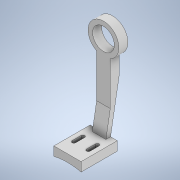
# Autodesk Inventor part: testBasePrint
Saved by Autodesk Inventor 2020.3 (Build 243373000, 373)
## iProperties
Created: 2020-06-03
Part Number: testBasePrint
Material: Generic
Document SubType Name: Modeling
Designer: robst
Density: 1 g/cm^3
Appearance: Default
Author: robst
Autodesk Inventor part; units mm, degrees
ref_plane "Work Plane3" through (19.05, 80.3219, 25.4) normal (0, 1, 0) x (-1, 0, 0)
ref_plane "Work Plane4" through (0, 228.9119, -25.0164) normal (0, 1, 0) x (-1, 0, 0)
sketch "Sketch1" plane through (0, 0, 0) normal (0, 0, 1) x (1, 0, 0)
  arc A0 (19.05, 80.3219) -> (-19.05, 80.3219) centre (0, 0) ccw
  line L0 (0, 0) -> (0, 152.4) construction
  line L1 (0, 93.0219) -> (19.05, 93.0219)
  line L2 (19.05, 93.0219) -> (19.05, 80.3219)
  line L3 (0, 93.0219) -> (-19.05, 93.0219)
  line L4 (-19.05, 93.0219) -> (-19.05, 80.3219)
  dimension "telescopeTubeDiameter" = 165.1
  dimension "d1" = 152.4
  dimension "d2" = 19.05
  dimension "d3" = 12.7
  constraints: 10 end point, 2 point on circle, 2 symmetric about line, 1 centre point, 1 coincident, 1 horizontal, 1 perpendicular, 1 point on line, 1 vertical
  measures "telescopeTubeDiameter" diameter of A0
  measures "d1" distance of L0.start L0.end
  measures "d2" distance of L1.start L1.end
  measures "d3" distance of L1.end L2.end
extrude "Extrusion1" add sketch "Sketch1" along normal mid plane 50.8
sketch "Sketch2" plane through (-19.05, 93.0219, 25.4) normal (0, 1, 0) x (1, 0, 0)
  line L0 (38.1, 0) -> (0, 0) construction
  line L1 (19.05, 0) -> (19.05, 50.8) construction
  line L2 (0, 50.8) -> (38.1, 50.8) construction
  line L3 (0, 50.8) -> (0, 0) construction
  line L4 (0, 25.4) -> (38.1, 25.4) construction
  line L5 (38.1, 50.8) -> (38.1, 0) construction
  line L6 (29.21, 19.05) -> (29.21, 31.75) construction
  line L7 (31.75, 19.05) -> (31.75, 31.75)
  line L8 (26.67, 31.75) -> (26.67, 19.05)
  arc A0 (26.67, 19.05) -> (31.75, 19.05) centre (29.21, 19.05) ccw
  arc A1 (31.75, 31.75) -> (26.67, 31.75) centre (29.21, 31.75) ccw
  point P0 (19.05, 25.4)
  point P1 (29.21, 25.4)
  dimension "d6" = 0
  dimension "d7" = 10.16
  dimension "d8" = 6.35
  dimension "d11" = 5.08
  constraints: 12 end point, 5 midpoint, 4 point on circle, 4 tangent, 2 centre point, 2 parallel
  measures "d6" distance from line of point (29.21, 25.4) L4
  measures "d7" distance between parallel lines of L6 L1
  measures "d8" distance of L6.end point (29.21, 25.4)
  measures "d11" distance between parallel lines of L7 L8
extrude "Extrusion2" cut sketch "Sketch2" against normal through all
mirror "Mirror1" about plane through (0, 0, 0) normal (1, 0, 0) of "Extrusion2"
sketch "Sketch3" plane through (0, 0, 0) normal (1, 0, 0) x (0, 1, 0)
  line L0 (93.0219, 25.4) -> (93.0219, -25.4) projected
  line L1 (80.3219, -25.4) -> (93.0219, -25.4) projected
  line L2 (162.8719, -25.4) -> (162.8719, -37.137) construction
  line L3 (93.0219, -25.4) -> (162.8719, -37.7164)
  line L4 (93.0219, -25.4) -> (162.8719, -25.4) construction
  line L5 (93.0219, -18.952) -> (162.8719, -31.2685)
  line L6 (162.8719, -31.2685) -> (162.8719, -37.7164)
  point P0 (0, 0)
  dimension "d13" = 69.85
  dimension "d14" = 10
  dimension "d15" = 6.35
  constraints: 10 end point, 2 point on line, 1 midpoint, 1 parallel, 1 perpendicular, 1 vertical
  measures "d13" distance of L0.end L2.start
  measures "d14" angle of L3 L4
  measures "d15" distance between parallel lines of L5 L3
extrude "Extrusion3" add sketch "Sketch3" along normal mid plane 19.05
ref_plane "Work Plane1" through (9.525, 162.8719, -37.7164) normal (0, 0, 1) x (1, 0, 0)
sketch "Sketch4" plane through (9.525, 162.8719, -37.7164) normal (0, 0, 1) x (1, 0, 0)
  line L0 (0, 0) -> (-19.05, 0) projected
  line L1 (-19.05, 0) -> (0, 0) construction
  line L2 (-9.525, 0) -> (-9.525, 50.8) construction
  circle A0 centre (-9.525, 44.45) radius 15.24
  arc A1 (0, 25.0747) -> (-19.05, 25.0747) centre (-9.525, 44.45) ccw
  line L3 (0, 0) -> (0, 25.0747)
  line L4 (-19.05, 0) -> (-19.05, 25.0747)
  point P0 (-9.525, -162.8719)
  dimension "d18" = 50.8
  dimension "d19" = 30.48
  dimension "d20" = 6.35
  dimension "d25" = 44.45
  constraints: 6 end point, 2 centre point, 2 point on circle, 2 vertical, 1 coincident, 1 midpoint, 1 parallel, 1 point on line
  measures "d18" distance of L2.start L2.end
  measures "d19" diameter of A0
  measures "d20" radial gap between concentric circles of A1 A0
  measures "d25" distance from line of A0.centre L0
extrude "Extrusion4" add sketch "Sketch4" along normal blind 12.7
sketch "Sketch7" plane through (0, 0, 0) normal (1, 0, 0) x (0, 1, 0)
  line L0 (93.0219, -18.952) -> (162.8719, -31.2685) projected
  line L1 (162.8719, -31.2685) -> (162.8719, -25.0164) projected
  line L2 (162.8719, -25.0164) -> (127.4148, -25.0164)
  line L3 (127.4148, -25.0164) -> (162.8719, -31.2685)
  line L4 (187.9465, -25.0164) -> (162.8719, -25.0164) projected
  line L5 (162.8719, -31.2685) -> (162.8719, -25.0164)
  point P0 (0, 0)
  constraints: 6 end point, 1 collinear, 1 horizontal, 1 point on line, 1 vertical
extrude "Extrusion5" add sketch "Sketch7" along normal mid plane 19.05
sketch "Sketch8" plane through (0, 0, 0) normal (1, 0, 0) x (0, 1, 0)
  line L0 (162.8719, 31.2685) -> (162.8719, 25.0164) projected
  line L1 (93.0219, 18.952) -> (162.8719, 31.2685) projected
  line L2 (162.8719, 25.0164) -> (127.4148, 25.0164)
  line L3 (127.4148, 25.0164) -> (162.8719, 31.2685)
  line L4 (162.8719, 31.2685) -> (162.8719, 25.0164)
  point P0 (0, 0)
  constraints: 6 end point, 1 collinear, 1 horizontal, 1 point on line
sketch "Sketch9" plane through (0, 0, 0) normal (1, 0, 0) x (0, 1, 0)
  line L0 (187.9465, 25.0164) -> (127.4148, 25.0164) projected
  line L1 (93.0219, -18.952) -> (93.0219, -25.4) projected
  line L2 (93.0219, 18.952) -> (93.0219, -18.952)
  line L3 (93.0219, -18.952) -> (127.4148, -25.0164) projected
  line L4 (93.0219, -18.952) -> (127.4148, -25.0164)
  line L5 (187.9465, -25.0164) -> (127.4148, -25.0164) projected
  line L6 (127.4148, -25.0164) -> (187.9465, -25.0164)
  line L7 (187.9465, -25.0164) -> (187.9465, 25.0164)
  line L8 (93.0219, 18.952) -> (127.4148, 25.0164) projected
  line L9 (187.9465, 25.0164) -> (127.4148, 25.0164)
  point P0 (0, 0)
  constraints: 10 end point, 2 collinear, 1 horizontal, 1 perpendicular, 1 vertical
sketch "Sketch14" plane through (0, 228.9119, -25.0164) normal (0, 1, 0) x (-1, 0, 0)
  circle A0 centre (0, -6.35) radius 2.0193
  line L0 (21.59, -12.7) -> (-21.59, -12.7) projected
  circle A1 centre (0, 56.3829) radius 2.0193
  line L1 (21.59, 62.7329) -> (-21.59, 62.7329) projected
  point P0 (0, 25.0164)
  point P1 (-9.525, -12.7)
  point P2 (9.525, -12.7)
  point P3 (-9.525, 62.7329)
  point P4 (9.525, 62.7329)
  dimension "d74" = 4.0386
  dimension "d75" = 6.35
  dimension "d76" = 6.35
  constraints: 2 centre point, 1 equal radius
  measures "d74" diameter of A0
  measures "d75" distance from line of A0.centre L0
  measures "d76" distance from line of A1.centre L1
sketch "Sketch16" plane through (0, 222.4275, -31.3664) normal (-1, 0, 0) x (0, 0, 1)
  line L0 (2.0193, 0) -> (2.0193, 6.4844)
  line L1 (2.0193, 6.4844) -> (1.4308, 6.4844)
  line L2 (1.4308, 6.4844) -> (1.4308, 0)
  line L3 (1.4308, 0) -> (2.0193, 0)
  line L4 (0, -171.8239) -> (0, 36.2042) projected
  constraints: 8 end point
sketch "Sketch15" plane through (0, 222.4275, -29.3471) normal (1, 0, 0) x (0, 1, 0)
  line L0 (-0.4631, -0.0403) -> (-0.397, -0.0403) construction
  line L1 (0.066, -0.5486) -> (-0.0001, -0.6756) construction
  line L2 (-0.7939, -0.6756) -> (-0.86, -0.5486) construction
  line L3 (-0.3308, -0.0403) -> (-0.397, 0.0868) construction
  line L4 (-0.397, 0.0868) -> (-0.4631, -0.0403) construction
  line L5 (-0.7939, -0.6756) -> (-0.7277, -0.5486) construction
  line L6 (-0.3308, -0.0403) -> (-0.0662, -0.5486)
  line L7 (-0.86, -0.5486) -> (-0.7277, -0.5486) construction
  arc A0 (-0.86, -0.5486) -> (-0.7939, -0.5887) centre (-0.7939, -0.5141) ccw construction
  line L8 (0.066, -0.5486) -> (-0.0662, -0.5486) construction
  line L9 (-0.7939, -0.6756) -> (-0.7939, -0.5486) construction
  line L10 (-0.0001, -0.6756) -> (-0.0001, -0.5486) construction
  line L11 (-0.397, 0.0868) -> (-0.397, -0.0002) construction
  line L12 (-0.7939, -0.5887) -> (-0.0001, -0.5887)
  arc A1 (-0.7939, -0.5887) -> (-0.7277, -0.5486) centre (-0.7939, -0.5141) ccw
  line L13 (-0.0662, -0.5486) -> (-0.0001, -0.6756) construction
  line L14 (-0.7277, -0.5486) -> (-0.4631, -0.0403)
  line L15 (-0.0001, -0.0002) -> (-0.0001, 0.0177)
  line L16 (-0.0001, 0.0177) -> (-0.0001, -0.0002)
  line L17 (-0.0001, -0.0002) -> (0.0334, -0.0002)
  arc A2 (-0.0662, -0.5486) -> (-0.0001, -0.5887) centre (-0.0001, -0.5141) ccw
  arc A3 (-0.0001, -0.5887) -> (0.066, -0.5486) centre (-0.0001, -0.5141) ccw construction
  arc A4 (-0.397, -0.0002) -> (-0.4631, -0.0403) centre (-0.397, -0.0747) ccw
  arc A5 (-0.3308, -0.0403) -> (-0.397, -0.0002) centre (-0.397, -0.0747) ccw
  line L18 (-0.397, -0.0002) -> (-0.397, -0.0403) construction
  line L19 (-0.397, -0.0403) -> (-0.3308, -0.0403) construction
  dimension "d94" = 55
  dimension "d95" = 0.1271
  dimension "d96" = 0.1271
  dimension "Sketch15_ThreadOffset" = 0
  dimension "Sketch15_MajorRadius" = 0.5885
  dimension "d99" = 0.7937
  dimension "Sketch15_MinorRadius" = 0
  constraints: 40 end point, 12 point on circle, 10 parallel, 8 tangent, 6 centre point, 6 collinear, 2 midpoint, 2 point on line, 1 horizontal, 1 perpendicular, 3 other
  measures "d94" angle of L6 L14
  measures "d95" distance of L3.end L0.end
  measures "d96" distance of L1.end L10.end
  measures "Sketch15_ThreadOffset" distance between parallel lines of L15 L10
  measures "Sketch15_MajorRadius" distance from line of L12 L15.start
  measures "d99" distance from line of L1.end L9
  measures "Sketch15_MinorRadius" distance edge to line of A5 L17
sketch "Sketch18" plane through (0, 222.4275, 31.3664) normal (-1, 0, 0) x (0, 0, 1)
  line L0 (2.0193, 0) -> (2.0193, 6.4844)
  line L1 (2.0193, 6.4844) -> (1.4308, 6.4844)
  line L2 (1.4308, 6.4844) -> (1.4308, 0)
  line L3 (1.4308, 0) -> (2.0193, 0)
  line L4 (0, -171.8765) -> (0, 36.5199) projected
  constraints: 8 end point
sketch "Sketch17" plane through (0, 222.4275, 33.3857) normal (1, 0, 0) x (0, 1, 0)
  line L0 (-0.4631, -0.0403) -> (-0.397, -0.0403) construction
  line L1 (0.066, -0.5486) -> (-0.0001, -0.6756) construction
  line L2 (-0.7939, -0.6756) -> (-0.86, -0.5486) construction
  line L3 (-0.3308, -0.0403) -> (-0.397, 0.0868) construction
  line L4 (-0.397, 0.0868) -> (-0.4631, -0.0403) construction
  line L5 (-0.7939, -0.6756) -> (-0.7277, -0.5486) construction
  line L6 (-0.3308, -0.0403) -> (-0.0662, -0.5486)
  line L7 (-0.86, -0.5486) -> (-0.7277, -0.5486) construction
  arc A0 (-0.86, -0.5486) -> (-0.7939, -0.5887) centre (-0.7939, -0.5141) ccw construction
  line L8 (0.066, -0.5486) -> (-0.0662, -0.5486) construction
  line L9 (-0.7939, -0.6756) -> (-0.7939, -0.5486) construction
  line L10 (-0.0001, -0.6756) -> (-0.0001, -0.5486) construction
  line L11 (-0.397, 0.0868) -> (-0.397, -0.0002) construction
  line L12 (-0.7939, -0.5887) -> (-0.0001, -0.5887)
  arc A1 (-0.7939, -0.5887) -> (-0.7277, -0.5486) centre (-0.7939, -0.5141) ccw
  line L13 (-0.0662, -0.5486) -> (-0.0001, -0.6756) construction
  line L14 (-0.7277, -0.5486) -> (-0.4631, -0.0403)
  line L15 (-0.0001, -0.0002) -> (-0.0001, 0.0177)
  line L16 (-0.0001, 0.0177) -> (-0.0001, -0.0002)
  line L17 (-0.0001, -0.0002) -> (0.0334, -0.0002)
  arc A2 (-0.0662, -0.5486) -> (-0.0001, -0.5887) centre (-0.0001, -0.5141) ccw
  arc A3 (-0.0001, -0.5887) -> (0.066, -0.5486) centre (-0.0001, -0.5141) ccw construction
  arc A4 (-0.397, -0.0002) -> (-0.4631, -0.0403) centre (-0.397, -0.0747) ccw
  arc A5 (-0.3308, -0.0403) -> (-0.397, -0.0002) centre (-0.397, -0.0747) ccw
  line L18 (-0.397, -0.0002) -> (-0.397, -0.0403) construction
  line L19 (-0.397, -0.0403) -> (-0.3308, -0.0403) construction
  dimension "d112" = 55
  dimension "d113" = 0.1271
  dimension "d114" = 0.1271
  dimension "Sketch17_ThreadOffset" = 0
  dimension "Sketch17_MajorRadius" = 0.5885
  dimension "d117" = 0.7937
  dimension "Sketch17_MinorRadius" = 0
  constraints: 40 end point, 12 point on circle, 10 parallel, 8 tangent, 6 centre point, 6 collinear, 2 midpoint, 2 point on line, 1 horizontal, 1 perpendicular, 3 other
  measures "d112" angle of L6 L14
  measures "d113" distance of L3.end L0.end
  measures "d114" distance of L1.end L10.end
  measures "Sketch17_ThreadOffset" distance between parallel lines of L15 L10
  measures "Sketch17_MajorRadius" distance from line of L12 L15.start
  measures "d117" distance from line of L1.end L9
  measures "Sketch17_MinorRadius" distance edge to line of A5 L17
sketch "Sketch20" plane through (13.0819, 199.769, -31.3664) normal (0.5, 0.866, 0) x (0, 0, 1)
  line L0 (2.0193, 0) -> (2.0193, 6.4844)
  line L1 (2.0193, 6.4844) -> (1.4308, 6.4844)
  line L2 (1.4308, 6.4844) -> (1.4308, 0)
  line L3 (1.4308, 0) -> (2.0193, 0)
  line L4 (0, -67.0949) -> (0, 89.4563) projected
  constraints: 8 end point
sketch "Sketch19" plane through (13.0819, 199.769, -29.3471) normal (-0.5, -0.866, 0) x (0.866, -0.5, 0)
  line L0 (-0.4631, -0.0403) -> (-0.397, -0.0403) construction
  line L1 (0.066, -0.5486) -> (-0.0001, -0.6756) construction
  line L2 (-0.7939, -0.6756) -> (-0.86, -0.5486) construction
  line L3 (-0.3308, -0.0403) -> (-0.397, 0.0868) construction
  line L4 (-0.397, 0.0868) -> (-0.4631, -0.0403) construction
  line L5 (-0.7939, -0.6756) -> (-0.7277, -0.5486) construction
  line L6 (-0.3308, -0.0403) -> (-0.0662, -0.5486)
  line L7 (-0.86, -0.5486) -> (-0.7277, -0.5486) construction
  arc A0 (-0.86, -0.5486) -> (-0.7939, -0.5887) centre (-0.7939, -0.5141) ccw construction
  line L8 (0.066, -0.5486) -> (-0.0662, -0.5486) construction
  line L9 (-0.7939, -0.6756) -> (-0.7939, -0.5486) construction
  line L10 (-0.0001, -0.6756) -> (-0.0001, -0.5486) construction
  line L11 (-0.397, 0.0868) -> (-0.397, -0.0002) construction
  line L12 (-0.7939, -0.5887) -> (-0.0001, -0.5887)
  arc A1 (-0.7939, -0.5887) -> (-0.7277, -0.5486) centre (-0.7939, -0.5141) ccw
  line L13 (-0.0662, -0.5486) -> (-0.0001, -0.6756) construction
  line L14 (-0.7277, -0.5486) -> (-0.4631, -0.0403)
  line L15 (-0.0001, -0.0002) -> (-0.0001, 0.0177)
  line L16 (-0.0001, 0.0177) -> (-0.0001, -0.0002)
  line L17 (-0.0001, -0.0002) -> (0.0334, -0.0002)
  arc A2 (-0.0662, -0.5486) -> (-0.0001, -0.5887) centre (-0.0001, -0.5141) ccw
  arc A3 (-0.0001, -0.5887) -> (0.066, -0.5486) centre (-0.0001, -0.5141) ccw construction
  arc A4 (-0.397, -0.0002) -> (-0.4631, -0.0403) centre (-0.397, -0.0747) ccw
  arc A5 (-0.3308, -0.0403) -> (-0.397, -0.0002) centre (-0.397, -0.0747) ccw
  line L18 (-0.397, -0.0002) -> (-0.397, -0.0403) construction
  line L19 (-0.397, -0.0403) -> (-0.3308, -0.0403) construction
  dimension "d130" = 55
  dimension "d131" = 0.1271
  dimension "d132" = 0.1271
  dimension "Sketch19_ThreadOffset" = 0
  dimension "Sketch19_MajorRadius" = 0.5885
  dimension "d135" = 0.7937
  dimension "Sketch19_MinorRadius" = 0
  constraints: 40 end point, 12 point on circle, 10 parallel, 8 tangent, 6 centre point, 6 collinear, 2 midpoint, 2 point on line, 1 horizontal, 1 perpendicular, 3 other
  measures "d130" angle of L6 L14
  measures "d131" distance of L3.end L0.end
  measures "d132" distance of L1.end L10.end
  measures "Sketch19_ThreadOffset" distance between parallel lines of L15 L10
  measures "Sketch19_MajorRadius" distance from line of L12 L15.start
  measures "d135" distance from line of L1.end L9
  measures "Sketch19_MinorRadius" distance edge to line of A5 L17
sketch "Sketch22" plane through (-13.0819, 199.769, -31.3664) normal (0.5, -0.866, 0) x (0, 0, 1)
  line L0 (2.0193, 0) -> (2.0193, 6.4844)
  line L1 (2.0193, 6.4844) -> (1.4308, 6.4844)
  line L2 (1.4308, 6.4844) -> (1.4308, 0)
  line L3 (1.4308, 0) -> (2.0193, 0)
  line L4 (0, -67.0949) -> (0, 89.4563) projected
  constraints: 8 end point
sketch "Sketch21" plane through (-13.0819, 199.769, -29.3471) normal (-0.5, 0.866, 0) x (-0.866, -0.5, 0)
  line L0 (-0.4631, -0.0403) -> (-0.397, -0.0403) construction
  line L1 (0.066, -0.5486) -> (-0.0001, -0.6756) construction
  line L2 (-0.7939, -0.6756) -> (-0.86, -0.5486) construction
  line L3 (-0.3308, -0.0403) -> (-0.397, 0.0868) construction
  line L4 (-0.397, 0.0868) -> (-0.4631, -0.0403) construction
  line L5 (-0.7939, -0.6756) -> (-0.7277, -0.5486) construction
  line L6 (-0.3308, -0.0403) -> (-0.0662, -0.5486)
  line L7 (-0.86, -0.5486) -> (-0.7277, -0.5486) construction
  arc A0 (-0.86, -0.5486) -> (-0.7939, -0.5887) centre (-0.7939, -0.5141) ccw construction
  line L8 (0.066, -0.5486) -> (-0.0662, -0.5486) construction
  line L9 (-0.7939, -0.6756) -> (-0.7939, -0.5486) construction
  line L10 (-0.0001, -0.6756) -> (-0.0001, -0.5486) construction
  line L11 (-0.397, 0.0868) -> (-0.397, -0.0002) construction
  line L12 (-0.7939, -0.5887) -> (-0.0001, -0.5887)
  arc A1 (-0.7939, -0.5887) -> (-0.7277, -0.5486) centre (-0.7939, -0.5141) ccw
  line L13 (-0.0662, -0.5486) -> (-0.0001, -0.6756) construction
  line L14 (-0.7277, -0.5486) -> (-0.4631, -0.0403)
  line L15 (-0.0001, -0.0002) -> (-0.0001, 0.0177)
  line L16 (-0.0001, 0.0177) -> (-0.0001, -0.0002)
  line L17 (-0.0001, -0.0002) -> (0.0334, -0.0002)
  arc A2 (-0.0662, -0.5486) -> (-0.0001, -0.5887) centre (-0.0001, -0.5141) ccw
  arc A3 (-0.0001, -0.5887) -> (0.066, -0.5486) centre (-0.0001, -0.5141) ccw construction
  arc A4 (-0.397, -0.0002) -> (-0.4631, -0.0403) centre (-0.397, -0.0747) ccw
  arc A5 (-0.3308, -0.0403) -> (-0.397, -0.0002) centre (-0.397, -0.0747) ccw
  line L18 (-0.397, -0.0002) -> (-0.397, -0.0403) construction
  line L19 (-0.397, -0.0403) -> (-0.3308, -0.0403) construction
  dimension "d148" = 55
  dimension "d149" = 0.1271
  dimension "d150" = 0.1271
  dimension "Sketch21_ThreadOffset" = 0
  dimension "Sketch21_MajorRadius" = 0.5885
  dimension "d153" = 0.7937
  dimension "Sketch21_MinorRadius" = 0
  constraints: 40 end point, 12 point on circle, 10 parallel, 8 tangent, 6 centre point, 6 collinear, 2 midpoint, 2 point on line, 1 horizontal, 1 perpendicular, 3 other
  measures "d148" angle of L6 L14
  measures "d149" distance of L3.end L0.end
  measures "d150" distance of L1.end L10.end
  measures "Sketch21_ThreadOffset" distance between parallel lines of L15 L10
  measures "Sketch21_MajorRadius" distance from line of L12 L15.start
  measures "d153" distance from line of L1.end L9
  measures "Sketch21_MinorRadius" distance edge to line of A5 L17
sketch "Sketch24" plane through (13.0819, 199.769, 31.3664) normal (0.5, 0.866, 0) x (0, 0, 1)
  line L0 (2.0193, 0) -> (2.0193, 6.4844)
  line L1 (2.0193, 6.4844) -> (1.4308, 6.4844)
  line L2 (1.4308, 6.4844) -> (1.4308, 0)
  line L3 (1.4308, 0) -> (2.0193, 0)
  line L4 (0, -67.0949) -> (0, 89.4563) projected
  constraints: 8 end point
sketch "Sketch23" plane through (13.0819, 199.769, 33.3857) normal (-0.5, -0.866, 0) x (0.866, -0.5, 0)
  line L0 (-0.4631, -0.0403) -> (-0.397, -0.0403) construction
  line L1 (0.066, -0.5486) -> (-0.0001, -0.6756) construction
  line L2 (-0.7939, -0.6756) -> (-0.86, -0.5486) construction
  line L3 (-0.3308, -0.0403) -> (-0.397, 0.0868) construction
  line L4 (-0.397, 0.0868) -> (-0.4631, -0.0403) construction
  line L5 (-0.7939, -0.6756) -> (-0.7277, -0.5486) construction
  line L6 (-0.3308, -0.0403) -> (-0.0662, -0.5486)
  line L7 (-0.86, -0.5486) -> (-0.7277, -0.5486) construction
  arc A0 (-0.86, -0.5486) -> (-0.7939, -0.5887) centre (-0.7939, -0.5141) ccw construction
  line L8 (0.066, -0.5486) -> (-0.0662, -0.5486) construction
  line L9 (-0.7939, -0.6756) -> (-0.7939, -0.5486) construction
  line L10 (-0.0001, -0.6756) -> (-0.0001, -0.5486) construction
  line L11 (-0.397, 0.0868) -> (-0.397, -0.0002) construction
  line L12 (-0.7939, -0.5887) -> (-0.0001, -0.5887)
  arc A1 (-0.7939, -0.5887) -> (-0.7277, -0.5486) centre (-0.7939, -0.5141) ccw
  line L13 (-0.0662, -0.5486) -> (-0.0001, -0.6756) construction
  line L14 (-0.7277, -0.5486) -> (-0.4631, -0.0403)
  line L15 (-0.0001, -0.0002) -> (-0.0001, 0.0177)
  line L16 (-0.0001, 0.0177) -> (-0.0001, -0.0002)
  line L17 (-0.0001, -0.0002) -> (0.0334, -0.0002)
  arc A2 (-0.0662, -0.5486) -> (-0.0001, -0.5887) centre (-0.0001, -0.5141) ccw
  arc A3 (-0.0001, -0.5887) -> (0.066, -0.5486) centre (-0.0001, -0.5141) ccw construction
  arc A4 (-0.397, -0.0002) -> (-0.4631, -0.0403) centre (-0.397, -0.0747) ccw
  arc A5 (-0.3308, -0.0403) -> (-0.397, -0.0002) centre (-0.397, -0.0747) ccw
  line L18 (-0.397, -0.0002) -> (-0.397, -0.0403) construction
  line L19 (-0.397, -0.0403) -> (-0.3308, -0.0403) construction
  dimension "d166" = 55
  dimension "d167" = 0.1271
  dimension "d168" = 0.1271
  dimension "Sketch23_ThreadOffset" = 0
  dimension "Sketch23_MajorRadius" = 0.5885
  dimension "d171" = 0.7937
  dimension "Sketch23_MinorRadius" = 0
  constraints: 40 end point, 12 point on circle, 10 parallel, 8 tangent, 6 centre point, 6 collinear, 2 midpoint, 2 point on line, 1 horizontal, 1 perpendicular, 3 other
  measures "d166" angle of L6 L14
  measures "d167" distance of L3.end L0.end
  measures "d168" distance of L1.end L10.end
  measures "Sketch23_ThreadOffset" distance between parallel lines of L15 L10
  measures "Sketch23_MajorRadius" distance from line of L12 L15.start
  measures "d171" distance from line of L1.end L9
  measures "Sketch23_MinorRadius" distance edge to line of A5 L17
sketch "Sketch26" plane through (-13.0819, 199.769, 31.3664) normal (0.5, -0.866, 0) x (0, 0, 1)
  line L0 (2.0193, 0) -> (2.0193, 6.4844)
  line L1 (2.0193, 6.4844) -> (1.4308, 6.4844)
  line L2 (1.4308, 6.4844) -> (1.4308, 0)
  line L3 (1.4308, 0) -> (2.0193, 0)
  line L4 (0, -67.0949) -> (0, 89.4563) projected
  constraints: 8 end point
sketch "Sketch25" plane through (-13.0819, 199.769, 33.3857) normal (-0.5, 0.866, 0) x (-0.866, -0.5, 0)
  line L0 (-0.4631, -0.0403) -> (-0.397, -0.0403) construction
  line L1 (0.066, -0.5486) -> (-0.0001, -0.6756) construction
  line L2 (-0.7939, -0.6756) -> (-0.86, -0.5486) construction
  line L3 (-0.3308, -0.0403) -> (-0.397, 0.0868) construction
  line L4 (-0.397, 0.0868) -> (-0.4631, -0.0403) construction
  line L5 (-0.7939, -0.6756) -> (-0.7277, -0.5486) construction
  line L6 (-0.3308, -0.0403) -> (-0.0662, -0.5486)
  line L7 (-0.86, -0.5486) -> (-0.7277, -0.5486) construction
  arc A0 (-0.86, -0.5486) -> (-0.7939, -0.5887) centre (-0.7939, -0.5141) ccw construction
  line L8 (0.066, -0.5486) -> (-0.0662, -0.5486) construction
  line L9 (-0.7939, -0.6756) -> (-0.7939, -0.5486) construction
  line L10 (-0.0001, -0.6756) -> (-0.0001, -0.5486) construction
  line L11 (-0.397, 0.0868) -> (-0.397, -0.0002) construction
  line L12 (-0.7939, -0.5887) -> (-0.0001, -0.5887)
  arc A1 (-0.7939, -0.5887) -> (-0.7277, -0.5486) centre (-0.7939, -0.5141) ccw
  line L13 (-0.0662, -0.5486) -> (-0.0001, -0.6756) construction
  line L14 (-0.7277, -0.5486) -> (-0.4631, -0.0403)
  line L15 (-0.0001, -0.0002) -> (-0.0001, 0.0177)
  line L16 (-0.0001, 0.0177) -> (-0.0001, -0.0002)
  line L17 (-0.0001, -0.0002) -> (0.0334, -0.0002)
  arc A2 (-0.0662, -0.5486) -> (-0.0001, -0.5887) centre (-0.0001, -0.5141) ccw
  arc A3 (-0.0001, -0.5887) -> (0.066, -0.5486) centre (-0.0001, -0.5141) ccw construction
  arc A4 (-0.397, -0.0002) -> (-0.4631, -0.0403) centre (-0.397, -0.0747) ccw
  arc A5 (-0.3308, -0.0403) -> (-0.397, -0.0002) centre (-0.397, -0.0747) ccw
  line L18 (-0.397, -0.0002) -> (-0.397, -0.0403) construction
  line L19 (-0.397, -0.0403) -> (-0.3308, -0.0403) construction
  dimension "d184" = 55
  dimension "d185" = 0.1271
  dimension "d186" = 0.1271
  dimension "Sketch25_ThreadOffset" = 0
  dimension "Sketch25_MajorRadius" = 0.5885
  dimension "d189" = 0.7937
  dimension "Sketch25_MinorRadius" = 0
  constraints: 40 end point, 12 point on circle, 10 parallel, 8 tangent, 6 centre point, 6 collinear, 2 midpoint, 2 point on line, 1 horizontal, 1 perpendicular, 3 other
  measures "d184" angle of L6 L14
  measures "d185" distance of L3.end L0.end
  measures "d186" distance of L1.end L10.end
  measures "Sketch25_ThreadOffset" distance between parallel lines of L15 L10
  measures "Sketch25_MajorRadius" distance from line of L12 L15.start
  measures "d189" distance from line of L1.end L9
  measures "Sketch25_MinorRadius" distance edge to line of A5 L17
equation "\"d94\" = d101"
equation "\"d95\" = 0.160083 * Sketch15_Pitch"
equation "\"d96\" = 0.160083 * Sketch15_Pitch"
equation "\"d99\" = Sketch15_Pitch"
equation "\"d112\" = d119"
equation "\"d113\" = 0.160083 * Sketch17_Pitch"
equation "\"d114\" = 0.160083 * Sketch17_Pitch"
equation "\"d117\" = Sketch17_Pitch"
equation "\"d130\" = d137"
equation "\"d131\" = 0.160083 * Sketch19_Pitch"
equation "\"d132\" = 0.160083 * Sketch19_Pitch"
equation "\"d135\" = Sketch19_Pitch"
equation "\"d148\" = d155"
equation "\"d149\" = 0.160083 * Sketch21_Pitch"
equation "\"d150\" = 0.160083 * Sketch21_Pitch"
equation "\"d153\" = Sketch21_Pitch"
equation "\"d166\" = d173"
equation "\"d167\" = 0.160083 * Sketch23_Pitch"
equation "\"d168\" = 0.160083 * Sketch23_Pitch"
equation "\"d171\" = Sketch23_Pitch"
equation "\"d184\" = d191"
equation "\"d185\" = 0.160083 * Sketch25_Pitch"
equation "\"d186\" = 0.160083 * Sketch25_Pitch"
equation "\"d189\" = Sketch25_Pitch"
equation "\"d62\" = 0.125 * Sketch12_Pitch"
equation "\"Sketch12_Pitch\" = 0.79375"
equation "\"d64\" = 60deg"
equation "\"d101\" = 55deg"
equation "\"Sketch15_Pitch\" = 0.79375"
equation "\"d119\" = 55deg"
equation "\"Sketch17_Pitch\" = 0.79375"
equation "\"d137\" = 55deg"
equation "\"Sketch19_Pitch\" = 0.79375"
equation "\"d155\" = 55deg"
equation "\"Sketch21_Pitch\" = 0.79375"
equation "\"d173\" = 55deg"
equation "\"Sketch23_Pitch\" = 0.79375"
equation "\"d191\" = 55deg"
equation "\"Sketch25_Pitch\" = 0.79375"
body "Solid1"
body "Solid3"
body "Solid4"
body "Solid5"
body "Solid6"
body "Solid7"
body "Solid8"
